Steper no cover v5 (Autodesk Fusion 360 design; units mm, degrees)
Autodesk Fusion 360 part; units mm, degrees
sketch "Sketch1" plane through (0, 0, 0) normal (0, 0, 1) x (1, 0, 0)
  line L0 (0, 0) -> (117.82, 0)
  line L1 (117.82, 0) -> (117.82, 72.6)
  line L2 (117.82, 72.6) -> (0, 72.6)
  line L3 (0, 72.6) -> (0, 0)
  circle A0 centre (10.6, 67.88) radius 1.4
  circle A1 centre (10.6, 4.78) radius 1.4
  circle A2 centre (105.7, 67.88) radius 1.4
  line L4 (10.6, 67.88) -> (10.6, 69.28) construction
  line L5 (105.7, 67.88) -> (105.7, 69.28) construction
  line L6 (10.6, 67.88) -> (9.2, 67.88) construction
  line L7 (105.7, 67.88) -> (107.1, 67.88) construction
  line L8 (10.6, 4.78) -> (10.6, 3.38) construction
  line L9 (10.6, 4.78) -> (9.2, 4.78) construction
  line L10 (10.6, 67.88) -> (105.7, 67.88) construction
  line L11 (10.6, 67.88) -> (10.6, 4.78) construction
  line L12 (0, 36.3) -> (117.82, 36.3) construction
  circle A3 centre (3, 36.3) radius 1.5
  circle A4 centre (115.12, 36.3) radius 1.5
  dimension "d1" = 117.82
  dimension "d2" = 72.6
  dimension "d3" = 2.8
  dimension "d4" = 2.8
  dimension "d6" = 2.8
  dimension "d18" = 95.1
  dimension "d19" = 63.1
  dimension "d20" = 4.72
  dimension "d21" = 10.6
  dimension "d22" = 3
  dimension "d23" = 3
  dimension "d24" = 2.7
  dimension "d25" = 3
  constraint horizontal L0
  constraint vertical L1
  constraint horizontal L2
  constraint vertical L3
  constraint coincident L0.start L3.end
  constraint coincident A0.centre L4.start
  constraint coincident A0 L4.end
  constraint perpendicular L2 L4
  constraint coincident A2.centre L5.start
  constraint coincident A2 L5.end
  constraint vertical L5
  constraint coincident A0 L6.end
  constraint perpendicular L4 L6
  constraint coincident A2 L7.end
  constraint perpendicular L5 L7
  constraint coincident A1.centre L8.start
  constraint coincident A1 L8.end
  constraint vertical L8
  constraint coincident A1 L9.end
  constraint perpendicular L8 L9
  constraint perpendicular L5 L10
  constraint perpendicular L9 L11
  constraint midpoint L3 L12.start
  constraint midpoint L1 L12.end
  constraint coincident L12 A3.centre
  constraint coincident L12 A4.centre
  measures "d1" distance of L0.start L0.end
  measures "d2" distance of L0.end L1.end
  measures "d3" diameter of A0
  measures "d4" diameter of A1
  measures "d6" diameter of A2
  measures "d18" distance of A0.centre A2.centre
  measures "d19" distance of A0.centre A1.centre
  measures "d20" distance of L2 A0.centre
  measures "d21" distance of L3 A0.centre
  measures "d22" diameter of A3
  measures "d23" diameter of A4
  measures "d24" distance of L1 A4.centre
  measures "d25" distance of L3 A3.centre
sketch "Sketch2" plane through (0, 0, 0) normal (0, 0, -1) x (1, 0, 0)
  circle A0 centre (10.6, -67.88) radius 1.4
  circle A1 centre (105.7, -67.88) radius 1.4
  circle A2 centre (10.6, -4.78) radius 1.4
  line L0 (0, 0) -> (0, -72.6)
  line L1 (0, -72.6) -> (117.82, -72.6)
  line L2 (117.82, -72.6) -> (117.82, 0)
  line L3 (117.82, 0) -> (0, 0)
  line L4 (117.82, -72.6) -> (0, 0) construction
  line L5 (0, -72.6) -> (117.82, 0) construction
  line L6 (88.1333, -48) -> (51.3806, -48)
  line L7 (51.3806, -48) -> (51.3806, -6)
  line L8 (51.3806, -6) -> (88.1333, -6)
  line L9 (88.1333, -6) -> (88.1333, -48)
  circle A3 centre (3, -36.3) radius 1.5
  circle A4 centre (115.12, -36.3) radius 1.5
  constraint coincident L1.end L2.start
  constraint coincident L0.start L3.end
  constraint coincident L2.end L3.start
  constraint coincident L0.end L1.start
  constraint horizontal L6
  constraint vertical L7
  constraint horizontal L8
  constraint vertical L9
sketch "Sketch3" plane through (0, 0, 1.5) normal (0, 0, 1) x (-1, 0, 0)
  circle A0 centre (-10.6, -67.88) radius 1.4
  circle A1 centre (-105.7, -67.88) radius 1.4
  circle A2 centre (-10.6, -4.78) radius 1.4
  circle A3 centre (-3, -36.3) radius 1.5
  circle A4 centre (-115.12, -36.3) radius 1.5
  line L0 (0, -72.6) -> (0, 0)
  line L1 (0, 0) -> (-117.82, 0)
  line L2 (-117.82, 0) -> (-117.82, -72.6)
  line L3 (-117.82, -72.6) -> (0, -72.6)
  line L4 (-6.41, -73) -> (-111.41, -73)
  line L5 (-111.41, -73) -> (-111.41, 0)
  line L6 (-111.41, 0) -> (-6.41, 0)
  line L7 (-6.41, 0) -> (-6.41, -73)
  line L8 (-6.41, -41.1844) -> (-0.01, -41.1844)
  line L9 (-0.01, -41.1844) -> (-0.01, -31.8156)
  line L10 (-0.01, -31.8156) -> (-6.41, -31.8156)
  line L11 (-111.41, -40.5951) -> (-117.27, -40.5951)
  line L12 (-117.27, -40.5951) -> (-117.27, -32.0049)
  line L13 (-117.27, -32.0049) -> (-111.41, -32.0049)
  line L14 (-117.27, -36.3) -> (-111.41, -36.3) construction
  line L15 (-0.01, -36.5) -> (-6.41, -36.5) construction
  line L16 (-58.91, 0) -> (-58.91, -72.6) construction
  point P0 (-115.12, -36.3)
  point P1 (-3, -36.5)
  dimension "d26" = 105
  dimension "d27" = 73
  dimension "d30" = 6.4
  dimension "d31" = 117.26
  constraint horizontal L4
  constraint vertical L5
  constraint vertical L7
  constraint coincident L7 L8.start
  constraint perpendicular L7 L8
  constraint perpendicular L8 L9
  constraint coincident L7 L10.end
  constraint perpendicular L7 L10
  constraint coincident L5 L11.start
  constraint perpendicular L2 L11
  constraint perpendicular L11 L12
  constraint coincident L5 L13.end
  constraint perpendicular L5 L13
  constraint coincident P0 A4.centre
  constraint midpoint L12 L14.start
  constraint coincident L5 L14.end
  constraint perpendicular L5 L14
  constraint midpoint L9 L15.start
  constraint midpoint L7 L15.end
  constraint perpendicular L7 L15
  constraint coincident P1 L15
  constraint coincident P0 L14
  constraint coincident L1 L6.end
  constraint midpoint L1 L16.start
  constraint midpoint L3 L16.end
  constraint symmetric L5 L7 L16
  measures "d26" distance of L5.end L6.end
  measures "d27" distance of L4.end L5.end
  measures "d30" distance of L8.start L8.end
  measures "d31" distance of L9 L12
extrude "Extrude3" add sketch "Sketch3" along normal blind 22 contours A0 | A1 | A2 | L1 L3 L5 L6 L7
extrude "Extrude4" add sketch "Sketch3" along normal blind 2 contours L7 L8 L9 L10 | L5 L11 L12 L13
chamfer "Chamfer1" distance 5 angle 45 3 edges at (6.41, 36.3, 23.5) (58.91, 72.6, 23.5) (111.41, 36.3, 23.5)
shell "Shell1" thickness 2 removed faces 1 at (43.0767, 0, 8.8333)
extrude "Extrude5" cut sketch "Sketch1" along normal blind 3.5 contours A0 | A1 | A2
equation "d4 = d3"
equation "d6 = d3"
equation "d18 = 92.3 mm + d3"
equation "d19 = 60.3 mm + d3"
